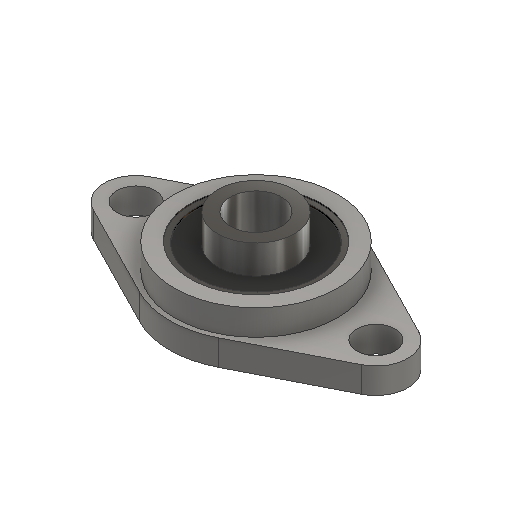
# Autodesk Inventor part: COTS_GENERIC_8mm_Dia_Ball_Screw_Top_Bearing_Block
Saved by Autodesk Inventor 2026.1 (Build 301233000, 233)
## iProperties
Created: 2016-03-27
Part Number: COTS_GENERIC_8mm_Dia_Ball_Screw_Top_Bearing_Block
Material: Tworzywo sztuczne LCP
Document SubType Name: Modeling
Designer: Andrzej
Density: 1.626 g/cm^3
Appearance: Brudny - ciemnobrązowy
Mass: 8.0515 g
Surface Area: 29.0636 cm^2
Volume: 4.95172 cm^3
Author: Andrzej
Autodesk Inventor part; units mm, degrees
ref_plane "YZ Plane" through (0, 0, 0) normal (1, 0, 0) x (0, 1, 0)
ref_plane "XZ Plane" through (0, 0, 0) normal (0, 1, 0) x (-1, 0, 0)
ref_plane "XY Plane" through (0, 0, 0) normal (0, 0, 1) x (1, 0, 0)
sketch "Szkic1" plane through (0, 0, 0) normal (0, 0, 1) x (1, 0, 0)
  arc A0 (21.0167, -4.4567) -> (21.0167, 4.4567) centre (18.75, 0) ccw
  arc A1 (-21.0167, 4.4567) -> (-21.0167, -4.4567) centre (-18.75, 0) ccw
  line L0 (6.12, -12.0331) -> (21.0167, -4.4567)
  line L1 (6.12, 12.0331) -> (21.0167, 4.4567)
  line L2 (-21.0167, 4.4567) -> (-6.12, 12.0331)
  line L3 (-21.0167, -4.4567) -> (-6.12, -12.0331)
  arc A2 (-6.12, -12.0331) -> (6.12, -12.0331) centre (0, 0) ccw
  arc A3 (6.12, 12.0331) -> (-6.12, 12.0331) centre (0, 0) ccw
  dimension "d3" = 10
  dimension "d4" = 10
  dimension "d5" = 37.5
  dimension "d6" = 18.75
  dimension "d7" = 0
  constraints: 8 end point, 8 point on circle, 8 tangent, 4 centre point, 1 coincident
  measures "d3" diameter of A0
  measures "d4" diameter of A1
  measures "d5" distance of A0.centre A1.centre
  measures "d6" distance of A0.centre point (0, 0)
  measures "d7" vertical distance of point (0, 0) A1.centre
extrude "Wyciągnięcie proste1" add sketch "Szkic1" along normal blind 4
sketch "Szkic2" plane through (0, 0, 4) normal (0, 0, 1) x (1, 0, 0)
  arc A0 (-21.0167, 4.4567) -> (-21.0167, -4.4567) centre (-18.75, 0) ccw projected
  line L0 (6.12, -12.0331) -> (21.0167, -4.4567) projected
  arc A1 (21.0167, -4.4567) -> (21.0167, 4.4567) centre (18.75, 0) ccw projected
  line L1 (21.0167, 4.4567) -> (6.12, 12.0331) projected
  arc A2 (6.12, 12.0331) -> (-6.12, 12.0331) centre (0, 0) ccw projected
  line L2 (-6.12, 12.0331) -> (-21.0167, 4.4567) projected
  arc A3 (-21.0167, 4.4567) -> (-21.0167, -4.4567) centre (-18.75, 0) ccw projected
  line L3 (-21.0167, -4.4567) -> (-6.12, -12.0331) projected
  arc A4 (-6.12, -12.0331) -> (6.12, -12.0331) centre (0, 0) ccw projected
  circle A5 centre (0, 0) radius 12.75
  dimension "d10" = 25.5
  constraints: 3 coincident, 1 centre point
  measures "d10" diameter of A5
extrude "Wyciągnięcie proste2" add sketch "Szkic2" along normal blind 4 contours A5
hole "Otwór1" at (18.75, 0, 4) at (-18.75, 0, 4) direction (0, 0, -1) diameter 6 end through all
sketch "Szkic3" plane through (0, 0, 8) normal (0, 0, 1) x (1, 0, 0)
  circle A0 centre (0, 0) radius 10.25
  circle A1 centre (0, 0) radius 9.45
  circle A2 centre (0, 0) radius 6
  circle A3 centre (0, 0) radius 4
  dimension "d20" = 20.5
  dimension "d21" = 0.8
  dimension "d22" = 12
  dimension "d23" = 2
  constraints: 4 centre point, 2 coincident
  measures "d20" diameter of A0
  measures "d21" radial gap between concentric circles of A0 A1
  measures "d22" diameter of A2
  measures "d23" radial gap between concentric circles of A2 A3
extrude "Wyciągnięcie proste3" cut sketch "Szkic3" against normal blind 0.2 contours A0
extrude "Wyciągnięcie proste4" cut sketch "Szkic3" against normal blind 0.5 contours A1
extrude "Wyciągnięcie proste5" cut sketch "Szkic3" against normal up to surface (8 mm away) contours A3
extrude "Wyciągnięcie proste6" add sketch "Szkic3" along normal blind 4 contours A2
equation "\"d6\" = 0.5 * d5"
